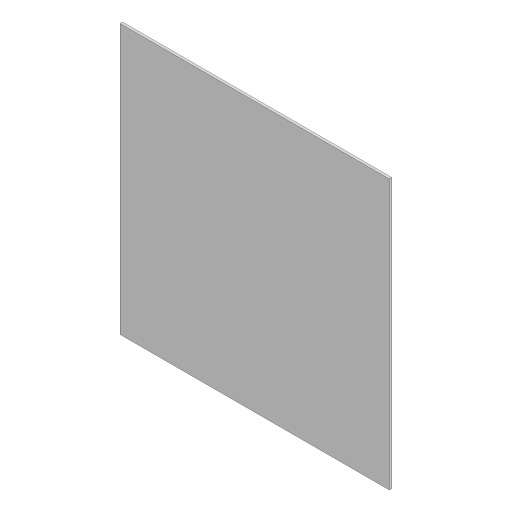
# Autodesk Inventor part: printer_base_plane
Saved by Autodesk Inventor 2024 (Build 280153000, 153)
## iProperties
Created: 2024-05-10
Part Number: printer_base_plane
Material: 一般
Document SubType Name: Modeling
Designer: admin
Density: 1 g/cm^3
Appearance: 預設
Author: admin
Autodesk Inventor part; units mm, degrees
ref_plane "YZ Plane" through (0, 0, 0) normal (1, 0, 0) x (0, 1, 0)
ref_plane "XZ Plane" through (0, 0, 0) normal (0, 1, 0) x (-1, 0, 0)
ref_plane "XY Plane" through (0, 0, 0) normal (0, 0, 1) x (1, 0, 0)
sketch "草圖1" plane through (0, 0, 0) normal (0, 0, 1) x (1, 0, 0)
  line L0 (-107.5, 107.5) -> (107.5, 107.5)
  line L1 (107.5, 107.5) -> (107.5, -107.5)
  line L2 (107.5, -107.5) -> (-107.5, -107.5)
  line L3 (-107.5, -107.5) -> (-107.5, 107.5)
  line L4 (-107.5, 107.5) -> (107.5, -107.5) construction
  line L5 (107.5, 107.5) -> (-107.5, -107.5) construction
  point P0 (0, 0)
  dimension "d0" = 215
  constraints: 12 end point, 2 midpoint, 2 parallel, 2 perpendicular, 1 horizontal
  measures "d0" distance of L0.start L0.end
extrude "擠出1" add sketch "草圖1" along normal blind 2
